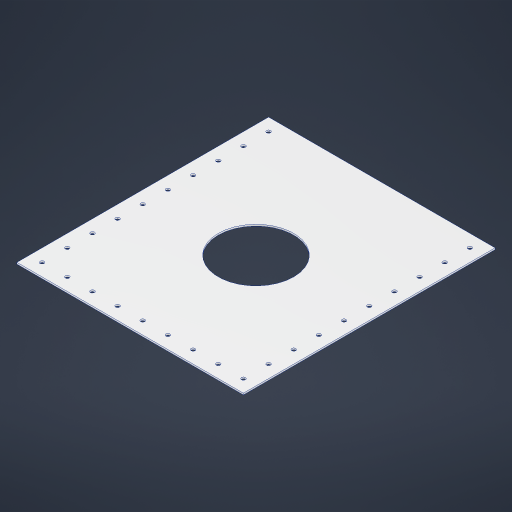
# Autodesk Inventor part: ArmPlate
Saved by Autodesk Inventor 2023 (Build 270158000, 158)
## iProperties
Created: 2023-01-19
Part Number: ArmPlate
Material: Aluminum 6061
Document SubType Name: Modeling
Designer: Nebil
Density: 2.7 g/cm^3
Appearance: Aluminum - Flat
Author: Nebil
Autodesk Inventor part; units mm, degrees
ref_plane "YZ Plane" through (0, 0, 0) normal (1, 0, 0) x (0, 1, 0)
ref_plane "XZ Plane" through (0, 0, 0) normal (0, 1, 0) x (-1, 0, 0)
ref_plane "XY Plane" through (0, 0, 0) normal (0, 0, 1) x (1, 0, 0)
sketch "Sketch1" plane through (0, 0, 0) normal (0, 1, 0) x (-1, 0, 0)
  line L0 (-114.3, 127) -> (114.3, 127)
  line L1 (114.3, 127) -> (114.3, -127)
  line L2 (114.3, -127) -> (-114.3, -127)
  line L3 (-114.3, -127) -> (-114.3, 127)
  line L4 (-114.3, 127) -> (114.3, -127) construction
  line L5 (114.3, 127) -> (-114.3, -127) construction
  circle A0 centre (101.6, 114.3) radius 2.0701
  circle A1 centre (101.6, 88.9) radius 2.0701
  circle A2 centre (101.6, 63.5) radius 2.0701
  circle A3 centre (101.6, 38.1) radius 2.0701
  circle A4 centre (101.6, 12.7) radius 2.0701
  circle A5 centre (101.6, -12.7) radius 2.0701
  circle A6 centre (101.6, -38.1) radius 2.0701
  circle A7 centre (101.6, -63.5) radius 2.0701
  circle A8 centre (101.6, -88.9) radius 2.0701
  circle A9 centre (101.6, -114.3) radius 2.0701
  circle A10 centre (76.2, 114.3) radius 2.0701
  circle A11 centre (50.8, 114.3) radius 2.0701
  circle A12 centre (25.4, 114.3) radius 2.0701
  circle A13 centre (0, 114.3) radius 2.0701
  circle A14 centre (-25.4, 114.3) radius 2.0701
  circle A15 centre (-50.8, 114.3) radius 2.0701
  circle A16 centre (-76.2, 114.3) radius 2.0701
  circle A17 centre (-101.6, 114.3) radius 2.0701
  circle A18 centre (0, 0) radius 38.1
  circle A19 centre (-101.6, 88.9) radius 2.0701
  circle A20 centre (-101.6, 63.5) radius 2.0701
  circle A21 centre (-101.6, 38.1) radius 2.0701
  circle A22 centre (-101.6, 12.7) radius 2.0701
  circle A23 centre (-101.6, -12.7) radius 2.0701
  circle A24 centre (-101.6, -38.1) radius 2.0701
  circle A25 centre (-101.6, -63.5) radius 2.0701
  circle A26 centre (-101.6, -88.9) radius 2.0701
  circle A27 centre (-101.6, -114.3) radius 2.0701
  dimension "d0" = 228.6
  dimension "d1" = 254
  dimension "d4" = 4.1402
  dimension "d5" = 12.7
  dimension "d6" = 12.7
  dimension "d9" = 25.4
  dimension "d16" = 25.4
  dimension "d28" = 76.2
  dimension "d31" = 25.4
  constraints: 28 centre point, 12 end point, 2 horizontal, 2 midpoint, 2 parallel, 2 vertical, 1 coincident, 1 perpendicular, 52 other
  measures "d0" distance of L1.end L2.end
  measures "d1" distance of L0.end L1.end
  measures "d4" diameter of A0
  measures "d5" distance from line of L1 A0.centre
  measures "d6" distance from line of L0 A0.centre
  measures "d9" distance of A0.centre A1.centre
  measures "d16" distance of A0.centre A10.centre
  measures "d28" diameter of A18
  measures "d31" distance of A17.centre A19.centre
extrude "Extrusion1" add sketch "Sketch1" along normal blind 1.5875
body "Solid1"
